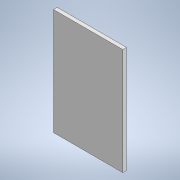
# Autodesk Inventor part: rear_case
Saved by Autodesk Inventor 2022.1 (Build 261234020, 234B)
## iProperties
Created: 2022-02-07
Part Number: rear_case
Material: Generic
Document SubType Name: Modeling
Designer: kee
Density: 1 g/cm^3
Appearance: Default
Mass: 77.905 g
Surface Area: 359.083 cm^2
Volume: 77.905 cm^3
Author: kee
Autodesk Inventor part; units mm, degrees
ref_plane "YZ Plane" through (0, 0, 0) normal (1, 0, 0) x (0, 1, 0)
ref_plane "XZ Plane" through (0, 0, 0) normal (0, 1, 0) x (-1, 0, 0)
ref_plane "XY Plane" through (0, 0, 0) normal (0, 0, 1) x (1, 0, 0)
sketch "Sketch3" plane through (0, 0, 0) normal (0, 0, 1) x (1, 0, 0)
  line L0 (42.5, 71.5) -> (-42.5, 71.5)
  line L1 (-46.5, 67.5) -> (-46.5, -67.5)
  line L2 (46.5, -67.5) -> (46.5, 67.5)
  line L3 (-42, 67) -> (42, 67) construction
  line L4 (42, 67) -> (42, -67) construction
  line L5 (42, -67) -> (-42, -67) construction
  line L6 (-42, -67) -> (-42, 67) construction
  arc A0 (-42.5, 71.5) -> (-46.5, 67.5) centre (-42.5, 67.5) ccw
  arc A1 (46.5, 67.5) -> (42.5, 71.5) centre (42.5, 67.5) ccw
  arc A2 (42.5, -71.5) -> (46.5, -67.5) centre (42.5, -67.5) ccw
  arc A3 (-46.5, -67.5) -> (-42.5, -71.5) centre (-42.5, -67.5) ccw
  line L7 (-39.5, -71.5) -> (-39.5, -74.9527)
  line L8 (-39.5, -74.9527) -> (39.5, -74.9527)
  line L9 (39.5, -74.9527) -> (39.5, -71.5)
  line L10 (-42.5, -71.5) -> (-39.5, -71.5)
  line L11 (39.5, -71.5) -> (42.5, -71.5)
  point P0 (0, 0)
  point P1 (46.5, 71.5)
  point P2 (-46.5, -71.5)
  point P3 (-46.5, 71.5)
  point P4 (46.5, -71.5)
  dimension "d7" = 93
  dimension "d9" = 46.5
  dimension "d10" = 71.5
  dimension "d11" = 84
  dimension "d12" = 134
  dimension "d13" = 42
  dimension "d14" = 67
  dimension "d15" = 4
  dimension "d16" = 4
  dimension "d17" = 79
  dimension "d18" = 39.5
  constraints: 24 end point, 10 tangent, 8 point on circle, 7 perpendicular, 6 point on line, 5 parallel, 4 centre point, 2 equal radius, 2 horizontal
  measures "d7" distance between parallel lines of L1 L2
  measures "d9" horizontal distance of point (0, 0) point (46.5, 71.5)
  measures "d10" vertical distance of point (-46.5, 71.5) point (0, 0)
  measures "d11" distance of L3.start L3.end
  measures "d12" distance of L3.end L4.end
  measures "d13" horizontal distance of point (0, 0) L3.start
  measures "d14" vertical distance of L3.end point (0, 0)
  measures "d15" radius of A0
  measures "d16" radius of A1
  measures "d17" distance of L7.end L8.end
  measures "d18" horizontal distance of point (0, 0) L7.end
extrude "Extrusion3" add sketch "Sketch3" along normal blind 5
sketch "Sketch4" plane through (0, 0, 0) normal (0, 0, -1) x (-1, 0, 0)
  line L0 (-39.5, -71.5) -> (39.5, -71.5)
  line L1 (39.5, -71.5) -> (39.5, -74.9527)
  line L2 (39.5, -74.9527) -> (-39.5, -74.9527)
  line L3 (-39.5, -74.9527) -> (-39.5, -71.5)
  point P0 (0, 0)
  constraints: 8 end point, 2 coincident, 2 parallel, 1 horizontal, 1 perpendicular
extrude "Extrusion4" add sketch "Sketch4" along normal blind 38
fillet "Fillet1" radius 3 2 edges at (39.5, -73.2264, -38) (-39.5, -73.2264, -38)
sketch "Sketch5" plane through (0, 0, 5) normal (0, 0, 1) x (1, 0, 0)
  line L0 (-42, 67) -> (42, 67) construction
  line L1 (42, 67) -> (42, -67) construction
  line L2 (42, -67) -> (-42, -67) construction
  line L3 (-42, -67) -> (-42, 67) construction
  point P0 (0, 0)
  dimension "d22" = 134
  dimension "d23" = 84
  dimension "d24" = 42
  dimension "d25" = 67
  constraints: 8 end point, 4 coincident, 2 parallel, 1 horizontal, 1 perpendicular
  measures "d22" distance of L0.end L1.end
  measures "d23" distance of L1.end L2.end
  measures "d24" horizontal distance of L1.end point (0, 0)
  measures "d25" vertical distance of L0.end point (0, 0)
hole "Hole1" at (-42, 67, 5) at (42, 67, 5) at (-42, -67, 5) at (42, -67, 5) direction (0, 0, -1) diameter 3 end through all counterbore diameter 4.6 counterbore depth 2.5
equation "\"d9\" = 0.5 * d7"
equation "\"d10\" = 0.5 * d8"
equation "\"d13\" = 0.5 * d11"
equation "\"d14\" = 0.5 * d12"
equation "\"d18\" = 0.5 * d17"
equation "\"d24\" = 0.5 * d23"
equation "\"d25\" = 0.5 * d22"
equation "\"d8\" = 143"
body "Solid2"
